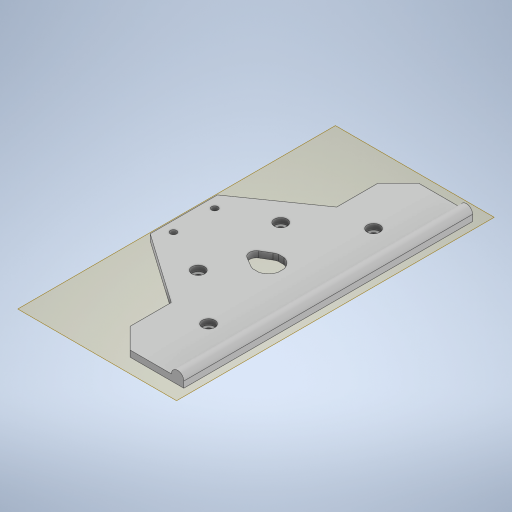
# Autodesk Inventor part: gripper_head 1b
Saved by Autodesk Inventor 2023 (Build 270158000, 158)
## iProperties
Created: 2024-07-03
Part Number: gripper_head 1b
Material: Generic
Document SubType Name: Modeling
Designer: Swoby
Density: 1 g/cm^3
Appearance: Default
Author: Swoby
Autodesk Inventor part; units mm, degrees
ref_plane "YZ Plane" through (0, 0, 0) normal (1, 0, 0) x (0, 1, 0)
ref_plane "XY Plane" through (0, 0, 0) normal (0, 0, 1) x (1, 0, 0)
sketch "Sketch1" plane through (0, 0, 0) normal (0, 0, 1) x (1, 0, 0)
  line L0 (-67, 3) -> (-67, -3)
  line L1 (-67, -3) -> (-3, -3)
  line L2 (-67, 3) -> (-3, 3)
  line L3 (0, -3) -> (0, 3) construction
  line L4 (3, -3) -> (3, 3)
  line L5 (-3, 3) -> (-3, -3)
  arc A0 (-3, -3) -> (3, -3) centre (0, -3) ccw
  arc A1 (3, 3) -> (-3, 3) centre (0, 3) ccw
  point P0 (0, 0)
  point P1 (-3, -3)
  dimension "d0" = 70
  dimension "d1" = 3
  dimension "d2" = 6
  dimension "d3" = 6
  constraints: 14 end point, 4 point on circle, 4 tangent, 2 centre point, 1 midpoint, 1 parallel, 1 perpendicular, 1 point on line, 1 vertical
  measures "d0" distance between parallel lines of L4 L0
  measures "d1" radius of A1
  measures "d2" distance between parallel lines of L1 L2
  measures "d3" distance of L3.start L3.end
extrude "Extrusion1" add sketch "Sketch1" along normal mid plane 140
sketch "Sketch2" plane through (-67, 3, 70) normal (0, 1, 0) x (1, 0, 0)
  line L0 (0, 0) -> (64, 0) projected
  line L1 (64, 0) -> (44, 0)
  line L2 (0, 140) -> (0, 0) projected
  line L3 (44, 0) -> (34, 10)
  line L4 (34, 10) -> (34, 29.9)
  line L5 (34, 29.9) -> (0, 53.7071)
  line L6 (0, 53.7071) -> (0, 86.2929)
  line L7 (0, 86.2929) -> (34, 110.1)
  line L8 (34, 110.1) -> (34, 130)
  line L9 (34, 130) -> (44, 140)
  line L10 (0, 140) -> (64, 140) projected
  line L11 (44, 140) -> (64, 140)
  line L12 (64, 140) -> (64, 0) projected
  point P0 (67, 70)
  dimension "d6" = 20
  dimension "d7" = 20
  dimension "d8" = 30
  dimension "d9" = 45
  dimension "d10" = 45
  dimension "d11" = 19.9
  dimension "d12" = 19.9
  dimension "d13" = 125
  dimension "d14" = 125
  constraints: 18 end point, 3 point on line, 2 collinear, 1 parallel, 1 vertical
  measures "d6" distance from line of L1.end L12
  measures "d7" distance from line of L12 L9.end
  measures "d8" distance between parallel lines of L12 L4
  measures "d9" angle of L0 L3
  measures "d10" angle of L10 L9
  measures "d11" distance of L3.end L4.end
  measures "d12" distance of L7.end L8.end
  measures "d13" angle of L5 L4
  measures "d14" angle of L7 L8
extrude "Extrusion2" cut sketch "Sketch2" against normal through all contours L2 L5 L4 L3 L0 | L2 L10 L9 L8 L7
sketch "Sketch3" plane through (-3, 3, 70) normal (0, 1, 0) x (1, 0, 0)
  circle A0 centre (-59, 80) radius 1.5
  circle A1 centre (-59, 60) radius 1.5
  line L0 (-64, 86.2929) -> (-64, 53.7071) projected
  line L1 (-59, 80) -> (-59, 60)
  point P0 (3, 70)
  point P1 (-64, 70)
  dimension "d17" = 3
  dimension "d18" = 3
  dimension "d19" = 20
  dimension "d20" = 10
  dimension "d21" = 5
  constraints: 2 centre point, 2 end point, 1 midpoint, 1 vertical
  measures "d17" diameter of A0
  measures "d18" diameter of A1
  measures "d19" distance of L1.end L1.start
  measures "d20" vertical distance of L1.start point (-64, 70)
  measures "d21" distance between parallel lines of L0 L1
extrude "Extrusion3" cut sketch "Sketch3" against normal through all
sketch "Sketch4" plane through (-3, 3, 70) normal (0, 1, 0) x (1, 0, 0)
  line L0 (-44.67, 64.05) -> (-12.45, 64.05)
  line L1 (-12.45, 64.05) -> (-12.45, 75.95)
  line L2 (-12.45, 75.95) -> (-44.67, 75.95)
  line L3 (-44.67, 75.95) -> (-44.67, 64.05)
  line L4 (-44.67, 64.05) -> (-12.45, 75.95) construction
  line L5 (-12.45, 64.05) -> (-44.67, 75.95) construction
  line L6 (6, 140) -> (6, 0) projected
  line L7 (6, 70) -> (-4, 70)
  line L8 (-40.17, 64.05) -> (-16.95, 64.05)
  line L9 (-16.95, 64.05) -> (-16.95, 75.95)
  line L10 (-16.95, 75.95) -> (-40.17, 75.95)
  line L11 (-40.17, 75.95) -> (-40.17, 64.05)
  line L12 (0, 140) -> (0, 0) projected
  line L13 (-44.87, 76.15) -> (-12.25, 76.15)
  line L14 (-12.25, 76.15) -> (-12.25, 63.85)
  line L15 (-12.25, 63.85) -> (-44.87, 63.85)
  line L16 (-44.87, 63.85) -> (-44.87, 76.15)
  line L17 (-47.37, 78.65) -> (-47.37, 61.35)
  line L18 (-9.75, 61.35) -> (-9.75, 78.65)
  circle A0 centre (-59, 80) radius 1.5 projected
  circle A1 centre (-59, 60) radius 1.5 projected
  line L19 (-47.37, 61.35) -> (-59.6538, 61.35)
  line L20 (-58.3462, 61.35) -> (-9.75, 61.35)
  line L21 (-9.75, 78.65) -> (-58.3462, 78.65)
  line L22 (-59.6538, 78.65) -> (-47.37, 78.65)
  circle A2 centre (-29, 70) radius 2.45
  point P0 (3, 70)
  point P1 (-28.56, 70)
  point P2 (-47.37, 78.65)
  point P3 (-47.37, 61.35)
  point P4 (-58.3462, 61.35)
  dimension "d24" = 32.22
  dimension "d25" = 11.9
  dimension "d26" = 4.5
  dimension "d27" = 4.5
  dimension "d30" = 0.2
  dimension "d34" = 2.5
  dimension "d35" = 2.5
  dimension "d36" = 2.5
  dimension "d37" = 2.5
  dimension "d51" = 29
  dimension "d52" = 12.05
  dimension "d53" = 4.9
  constraints: 42 end point, 11 parallel, 5 perpendicular, 5 point on line, 4 point on circle, 3 horizontal, 3 midpoint, 2 collinear, 1 centre point, 3 other
  measures "d24" distance of L1.end L2.end
  measures "d25" distance of L0.end L1.end
  measures "d26" distance between parallel lines of L3 L11
  measures "d27" distance between parallel lines of L1 L9
  measures "d30" distance between parallel lines of L2 L13
  measures "d34" distance between parallel lines of L17 L16
  measures "d35" distance between parallel lines of L18 L14
  measures "d36" distance between parallel lines of L13 L21
  measures "d37" distance between parallel lines of L20 L15
  measures "d51" distance from line of L12 A2.centre
  measures "d52" distance from line of L9 A2.centre
  measures "d53" diameter of A2
extrude "Extrusion4" add sketch "Sketch4" against normal blind 15 contours L3 L2 L11 L0 | L11 L2 L9 L0 | L9 L2 L1 L0 | L13 L14 L15 L16 | L21 L18 L20 L17 | A2
sketch "Sketch5" plane through (-3, -12, 70) normal (0, -1, 0) x (1, 0, 0)
  circle A0 centre (-59, -80) radius 1.5 projected
  circle A1 centre (-59, -60) radius 1.5 projected
  line L0 (-30, -110.1) -> (-64, -86.2929) projected
  line L1 (-64, -86.2929) -> (-64, -53.7071) projected
  line L2 (-64, -53.7071) -> (-30, -29.9) projected
  line L3 (-30, -29.9) -> (-30, -10) projected
  line L4 (-30, -10) -> (-20, 0) projected
  line L5 (0, 0) -> (-20, 0) projected
  line L6 (0, -140) -> (0, 0) projected
  line L7 (-20, -140) -> (0, -140) projected
  line L8 (-20, -140) -> (-30, -130) projected
  line L9 (-30, -130) -> (-30, -110.1) projected
  line L10 (-12.45, -75.95) -> (-44.67, -75.95) projected
  line L11 (-16.95, -64.05) -> (-16.95, -75.95) projected
  line L12 (-44.87, -76.15) -> (-12.25, -76.15) projected
  line L13 (-12.25, -76.15) -> (-12.25, -63.85) projected
  line L14 (-12.45, -64.05) -> (-12.45, -75.95) projected
  line L15 (-44.67, -64.05) -> (-12.45, -64.05) projected
  line L16 (-12.25, -63.85) -> (-44.87, -63.85) projected
  line L17 (-44.87, -63.85) -> (-44.87, -76.15) projected
  line L18 (-44.67, -75.95) -> (-44.67, -64.05) projected
  line L19 (-44.67, -64.05) -> (-12.45, -75.95) construction
  line L20 (-40.17, -75.95) -> (-40.17, -64.05) projected
  line L21 (-40.17, -75.95) -> (-40.17, -76.15)
  line L22 (-40.17, -64.05) -> (-40.17, -63.85)
  line L23 (-16.95, -76.15) -> (-16.95, -75.95)
  line L24 (-16.95, -64.05) -> (-16.95, -63.85)
  point P0 (3, -70)
  constraints: 8 end point, 7 point on line, 1 collinear
extrude "Extrusion5" cut sketch "Sketch5" against normal blind 7 contours L14 L15 L24 L16 L13 L12 L23 L10 | L10 L11 L15 L14 | L23 L12 L21 L10 | L10 L20 L15 L11 | L21 L12 L17 L16 L22 L15 L18 L10 | L10 L18 L15 L20 | L15 L22 L16 L24
sketch "Sketch6" plane through (-3, -5, 70) normal (0, -1, 0) x (1, 0, 0)
  line L0 (-16.95, -64.05) -> (-16.95, -75.95) construction
  line L1 (-12.45, -64.05) -> (-44.67, -75.95) construction
  line L2 (-40.17, -75.95) -> (-40.17, -64.05) construction
  line L3 (-12.25, -63.85) -> (-12.25, -76.15) projected
  line L4 (-44.87, -63.85) -> (-12.25, -63.85) projected
  line L5 (-44.87, -76.15) -> (-44.87, -63.85) projected
  line L6 (-12.25, -76.15) -> (-44.87, -76.15) projected
  line L7 (-16.95, -64.05) -> (-16.95, -63.85)
  line L8 (-44.87, -63.85) -> (-12.25, -63.85) projected
  line L9 (-16.95, -75.95) -> (-16.95, -76.15)
  line L10 (-40.17, -76.15) -> (-40.17, -75.95)
  line L11 (-40.17, -64.05) -> (-40.17, -63.85)
  line L12 (-40.32, -76.15) -> (-40.32, -63.85)
  line L13 (-16.8, -76.15) -> (-16.8, -63.85)
  line L14 (-40.32, -76.15) -> (-16.8, -76.15)
  line L15 (-16.8, -76.15) -> (-16.8, -63.85)
  line L16 (-16.8, -63.85) -> (-40.32, -63.85)
  line L17 (-40.32, -63.85) -> (-40.32, -76.15)
  point P0 (3, -70)
  dimension "d40" = 0.15
  dimension "d41" = 0.15
  constraints: 20 end point, 10 point on line, 4 parallel, 3 perpendicular, 1 horizontal
  measures "d40" distance between parallel lines of L2 L12
  measures "d41" distance between parallel lines of L13 L0
extrude "Extrusion6" cut sketch "Sketch6" against normal blind 5 contours L13 L6 L12 L4
sketch "Sketch7" plane through (-3, 0, 70) normal (0, -1, 0) x (1, 0, 0)
  line L0 (-16.8, -63.85) -> (-16.8, -76.15) projected
  line L1 (-16.8, -70) -> (-21, -70)
  circle A0 centre (-22.95, -70) radius 6.15 construction
  line L2 (-44.87, -63.85) -> (-12.25, -63.85) projected
  arc A1 (-24.3166, -63.85) -> (-24.3166, -76.15) centre (-22.95, -70) ccw
  circle A2 centre (-28.8, -70) radius 3 construction
  line L3 (-24.3166, -63.85) -> (-30.3313, -67.4202) construction
  line L4 (-30.3313, -72.5798) -> (-24.3166, -76.15) construction
  line L5 (-12.25, -76.15) -> (-44.87, -76.15) projected
  arc A3 (-21.5834, -63.85) -> (-24.3166, -63.85) centre (-22.95, -70) ccw construction
  arc A4 (-21.5834, -76.15) -> (-16.8, -71.3666) centre (-22.95, -70) ccw
  arc A5 (-24.3166, -76.15) -> (-21.5834, -76.15) centre (-22.95, -70) ccw construction
  arc A6 (-16.8, -71.3666) -> (-16.8, -68.6334) centre (-22.95, -70) ccw construction
  arc A7 (-16.8, -68.6334) -> (-21.5834, -63.85) centre (-22.95, -70) ccw
  line L6 (-26.1657, -64.5825) -> (-30.4916, -67.1503)
  arc A8 (-28.169, -66.7467) -> (-28.3286, -66.7197) centre (-28.8, -70) ccw
  arc A9 (-30.4916, -67.1503) -> (-30.4916, -72.8497) centre (-28.8, -70) ccw
  line L7 (-30.4916, -72.8497) -> (-26.1657, -75.4175)
  point P0 (3, -70)
  dimension "d44" = 0.15
  dimension "d45" = 6
  dimension "d46" = 12
  constraints: 22 point on circle, 10 end point, 9 centre point, 8 point on line, 5 tangent, 2 midpoint, 2 parallel, 1 horizontal, 1 perpendicular, 1 vertical, 3 other
  measures "d45" diameter of A2
  measures "d46" distance of A2.centre point (-16.8, -70)
extrude "Extrusion7" cut sketch "Sketch7" against normal through all contours L0 A4 L5 A1 L2 A7 | A1 L7 A9 L6
fillet "Fillet1" radius 2 4 edges at (-12.75, -7.5, -8.65) (-50.37, -7.5, -8.65) (-50.37, -7.5, 8.65) (-12.75, -7.5, 8.65)
sketch "Sketch8" plane through (-3, -3, -70) normal (0, -1, 0) x (1, 0, 0)
  circle A0 centre (-12, 110) radius 1.5
  circle A1 centre (-12, 30) radius 1.5
  circle A2 centre (-37, 50) radius 1.5
  circle A3 centre (-37, 90) radius 1.5
  line L0 (-12, 110) -> (-12, 30) construction
  line L1 (-37, 90) -> (-37, 50) construction
  line L2 (6, 0) -> (6, 140) projected
  line L3 (-64, 53.7071) -> (-64, 86.2929) projected
  line L4 (-64, 70) -> (6, 70) construction
  point P0 (3, 70)
  point P1 (-12, 70)
  point P2 (-37, 70)
  dimension "d54" = 3
  dimension "d55" = 3
  dimension "d56" = 18
  dimension "d57" = 25
  dimension "d58" = 80
  dimension "d59" = 3
  dimension "d60" = 40
  dimension "d61" = 3
  constraints: 6 end point, 4 centre point, 4 midpoint, 2 parallel, 2 point on line, 2 vertical
  measures "d54" diameter of A0
  measures "d55" diameter of A2
  measures "d56" distance between parallel lines of L2 L0
  measures "d57" distance between parallel lines of L1 L0
  measures "d58" distance of L0.end L0.start
  measures "d59" diameter of A1
  measures "d60" distance of L1.end L1.start
  measures "d61" diameter of A3
extrude "Extrusion8" cut sketch "Sketch8" along normal through all both and the other way through all
sketch "Sketch9" plane through (-3, 3, 70) normal (0, 1, 0) x (1, 0, 0)
  circle A0 centre (-12, 110) radius 1.5 projected
  circle A1 centre (-37, 90) radius 1.5 projected
  circle A2 centre (-37, 50) radius 1.5 projected
  circle A3 centre (-12, 30) radius 1.5 projected
  circle A4 centre (-12, 110) radius 3.05
  circle A5 centre (-12, 30) radius 3.05
  circle A6 centre (-37, 90) radius 3.05
  circle A7 centre (-37, 50) radius 1.5 projected
  circle A8 centre (-37, 50) radius 3.05
  point P0 (3, 70)
  dimension "d64" = 6.1
  dimension "d65" = 6.1
  dimension "d66" = 6.1
  dimension "d67" = 6.1
  constraints: 4 centre point, 4 coincident
  measures "d64" diameter of A4
  measures "d65" diameter of A5
  measures "d66" diameter of A6
  measures "d67" diameter of A8
extrude "Extrusion9" cut sketch "Sketch9" against normal blind 2.7 contours A0 | A1 | A2 | A3 | A4 | A5 | A6 | A8
sketch "Sketch10" plane through (-3, -3, -70) normal (0, -1, 0) x (1, 0, 0)
  circle A0 centre (-37, 50) radius 1.5 projected
  circle A1 centre (-37, 90) radius 1.5 projected
  circle A2 centre (-12, 110) radius 1.5 projected
  line L0 (-38.6454, 52.85) -> (-35.3546, 52.85)
  line L1 (-35.3546, 52.85) -> (-33.7091, 50)
  line L2 (-33.7091, 50) -> (-35.3546, 47.15)
  line L3 (-35.3546, 47.15) -> (-38.6454, 47.15)
  line L4 (-38.6454, 47.15) -> (-40.2909, 50)
  line L5 (-40.2909, 50) -> (-38.6454, 52.85)
  line L6 (-38.6454, 92.85) -> (-35.3546, 92.85)
  line L7 (-35.3546, 92.85) -> (-33.7091, 90)
  line L8 (-33.7091, 90) -> (-35.3546, 87.15)
  line L9 (-35.3546, 87.15) -> (-38.6454, 87.15)
  line L10 (-38.6454, 87.15) -> (-40.2909, 90)
  line L11 (-40.2909, 90) -> (-38.6454, 92.85)
  line L12 (-13.6454, 112.85) -> (-10.3546, 112.85)
  line L13 (-10.3546, 112.85) -> (-8.7091, 110)
  line L14 (-8.7091, 110) -> (-10.3546, 107.15)
  line L15 (-10.3546, 107.15) -> (-13.6454, 107.15)
  line L16 (-13.6454, 107.15) -> (-15.2909, 110)
  line L17 (-15.2909, 110) -> (-13.6454, 112.85)
  line L18 (-20, 140) -> (0, 140) projected
  line L19 (-10.3546, 32.85) -> (-8.7091, 30)
  line L20 (-8.7091, 30) -> (-10.3546, 27.15)
  line L21 (-10.3546, 27.15) -> (-13.6454, 27.15)
  line L22 (-13.6454, 27.15) -> (-15.2909, 30)
  line L23 (-15.2909, 30) -> (-13.6454, 32.85)
  line L24 (-13.6454, 32.85) -> (-10.3546, 32.85)
  point P0 (3, 70)
  point P1 (-12, 30)
  point P2 (-12, 30)
  point P3 (-37, 52.85)
  point P4 (-37, 47.15)
  dimension "d70" = 5.7
  dimension "d71" = 5.7
  dimension "d72" = 5.7
  dimension "d73" = 5.7
  constraints: 48 end point, 4 coincident, 4 parallel, 2 midpoint, 52 other
  measures "d70" distance between parallel lines of L24 L21
  measures "d71" distance of point (-37, 52.85) point (-37, 47.15)
  measures "d72" distance between parallel lines of L6 L9
  measures "d73" distance between parallel lines of L12 L15
extrude "Extrusion10" cut sketch "Sketch10" against normal blind 2.5
split "Split1" plane through (0, 0, 0) removes the side toward (0, -1, 0)
sketch "Sketch11" plane through (-3, 0, 70) normal (0, -1, 0) x (1, 0, 0)
  circle A0 centre (-14.81, -70) radius 0.55
  circle A1 centre (-42.31, -70) radius 0.55
  line L0 (-14.81, -70) -> (-42.31, -70)
  line L1 (-16.8, -71.3666) -> (-16.8, -68.6334) projected
  line L2 (6, 0) -> (6, -140) projected
  point P0 (3, -70)
  point P1 (-16.8, -70)
  dimension "d76" = 1.1
  dimension "d77" = 1.1
  dimension "d78" = 27.5
  dimension "d79" = 20.81
  constraints: 2 centre point, 2 end point, 1 horizontal, 1 midpoint, 1 point on line
  measures "d76" diameter of A0
  measures "d77" diameter of A1
  measures "d78" distance of L0.start L0.end
  measures "d79" distance from line of L2 L0.start
extrude "Extrusion11" cut sketch "Sketch11" against normal blind 1
chamfer "Chamfer1" distance 0.5 angle 45 2 edges at (-18.36, 1, 0) (-45.86, 1, 0)
equation "\"d7\" = d6"
equation "\"d10\" = d9"
equation "\"d12\" = d11"
equation "\"d14\" = d13"
equation "\"d27\" = d26"
equation "\"d34\" = d36"
equation "\"d35\" = d36"
equation "\"d37\" = d36"
equation "\"d71\" = d70"
equation "\"d72\" = d70"
equation "\"d73\" = d70"
body "Solid1"
